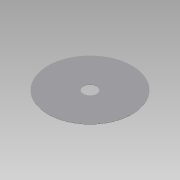
# Autodesk Inventor part: pig_butt_holder
Saved by Autodesk Inventor 2015 (Build 190159000, 159)
## iProperties
Created: 2016-05-01
Part Number: pig_butt_holder
Material: Generic
Document SubType Name: Modeling
Designer: Luke Good
Density: 1 g/cm^3
Appearance: Default
Author: Luke Good
Autodesk Inventor part; units mm, degrees
ref_plane "YZ Plane" through (0, 0, 0) normal (1, 0, 0) x (0, 1, 0)
ref_plane "XZ Plane" through (0, 0, 0) normal (0, 1, 0) x (-1, 0, 0)
ref_plane "XY Plane" through (0, 0, 0) normal (0, 0, 1) x (1, 0, 0)
sketch "Sketch1" plane through (0, 0, 0) normal (0, 1, 0) x (-1, 0, 0)
  arc A0 (62.2165, 72.7223) -> (87.0556, 72.7223) centre (74.6361, 61.0876) ccw
  arc A1 (62.2165, 72.7223) -> (87.0556, 72.7223) centre (74.6361, 61.0876) ccw
  arc A2 (87.0556, 72.7223) -> (62.2165, 72.7223) centre (74.6361, 61.0876) ccw
  circle A3 centre (74.6361, 61.0876) radius 106.1502
  point P0 (0, 0)
  point P1 (74.6361, 0)
  point P2 (0, 72.7223)
  point P3 (149.2721, 72.7223)
  point P4 (0, 0)
  dimension "d2" = 17.018
  constraints: 6 point on circle, 4 centre point, 2 coincident, 1 concentric
  measures "d2" radius of A0
extrude "Extrusion1" add sketch "Sketch1" along normal blind 0.508
body "Solid1"
